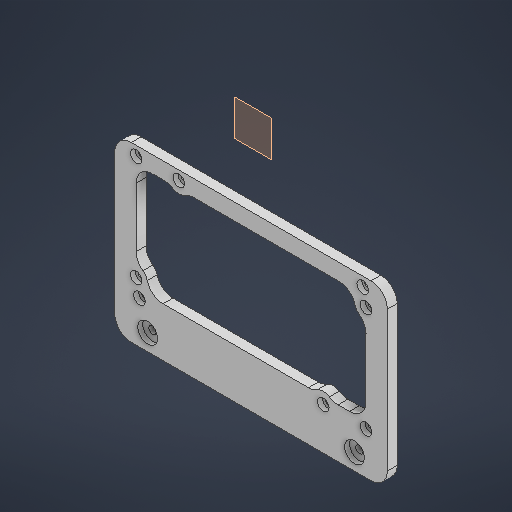
# Autodesk Inventor part: atx_power_holder
Saved by Autodesk Inventor 2026.2 (Build 302298010, 298A)
## iProperties
Created: 2025-02-06
Part Number: atx_power_holder
Material: 一般
Document SubType Name: Modeling
Designer: gisen
Density: 1 g/cm^3
Appearance: 既定
Author: gisen
Autodesk Inventor part; units mm, degrees
ref_plane "YZ Plane" through (0, 0, 0) normal (1, 0, 0) x (0, 1, 0)
ref_plane "XZ Plane" through (0, 0, 0) normal (0, 1, 0) x (-1, 0, 0)
ref_plane "XY Plane" through (0, 0, 0) normal (0, 0, 1) x (1, 0, 0)
sketch "スケッチ1" plane through (0, 0, 0) normal (0, 0, 1) x (1, 0, 0)
  circle A0 centre (44, 4.4) radius 1.25 construction
  circle A1 centre (68, 78.4) radius 1.25 construction
  circle A2 centre (-70, 78.4) radius 1.25 construction
  circle A3 centre (-70, 14.4) radius 1.25 construction
  arc A4 (22.159, 26.4069) -> (22.159, 19.1931) centre (24.5, 22.8) ccw construction
  line L0 (22.159, 26.4069) -> (30.5, 31.8205) construction
  line L1 (30.5, 13.7795) -> (22.159, 19.1931) construction
  line L2 (58.5, 31.8205) -> (66.841, 26.4069) construction
  arc A5 (66.841, 19.1931) -> (66.841, 26.4069) centre (64.5, 22.8) ccw construction
  line L3 (58.5, 13.7795) -> (66.841, 19.1931) construction
  line L4 (35.3264, 11.8) -> (53.6736, 11.8) construction
  line L5 (73.8, 84.2) -> (-73.8, 84.2) construction
  line L6 (75, 83) -> (75, 9.6971) construction
  line L7 (-75, 5.3) -> (-75, 0) construction
  line L8 (75, 0) -> (75, 5.3) construction
  line L9 (-75, 84.2) -> (75, 84.2) construction
  line L10 (75, 84.2) -> (75, -1.2) construction
  line L11 (75, -1.2) -> (-75, -1.2) construction
  line L12 (-75, -1.2) -> (-75, 84.2) construction
  line L13 (-73, -1.2) -> (73, -1.2) construction
  line L14 (75, 84.2) -> (-75, -1.2) construction
  circle A6 centre (-70, 78.4) radius 1.7
  circle A7 centre (-70, 14.4) radius 1.7
  circle A8 centre (44, 4.4) radius 1.7
  circle A9 centre (68, 78.4) radius 1.7
  circle A10 centre (-70, 78.4) radius 7 construction
  circle A11 centre (-70, 14.4) radius 7 construction
  circle A12 centre (44, 4.4) radius 7 construction
  circle A13 centre (68, 78.4) radius 7 construction
  circle A14 centre (70, 4.6) radius 7 construction
  circle A15 centre (70, 4.6) radius 1.7
  circle A16 centre (70, 68.6) radius 7 construction
  circle A17 centre (70, 68.6) radius 1.7
  circle A18 centre (-44, 78.6) radius 7 construction
  circle A19 centre (-44, 78.6) radius 1.7
  circle A20 centre (-68, 4.6) radius 7 construction
  circle A21 centre (-68, 4.6) radius 1.7
  line L15 (-70, 74.2) -> (70, 74.2) construction
  line L16 (70, 74.2) -> (70, 8.8) construction
  line L17 (70, 8.8) -> (-70, 8.8) construction
  line L18 (-70, 8.8) -> (-70, 74.2) construction
  line L19 (90, 128.8) -> (-75, 128.8)
  line L20 (-75, 128.8) -> (-75, -1.2)
  line L21 (-75, -1.2) -> (90, -1.2)
  line L22 (90, -1.2) -> (90, 128.8)
  line L23 (-70, 71.4) -> (-70, 21.4)
  line L24 (-64.4, 74.2) -> (-49.4443, 74.2)
  line L25 (-38.5557, 74.2) -> (62.4, 74.2)
  line L26 (70, 61.6) -> (70, 11.6)
  line L27 (64.4, 8.8) -> (49.4443, 8.8)
  line L28 (38.5557, 8.8) -> (-62.4, 8.8)
  arc A22 (-64.201, 10.4794) -> (-70, 21.4) centre (-70, 14.4) ccw
  arc A23 (-62.4, 8.8) -> (-64.201, 10.4794) centre (-68, 4.6) ccw
  arc A24 (-70, 71.4) -> (-64.4, 74.2) centre (-70, 78.4) ccw
  arc A25 (-49.4443, 74.2) -> (-38.5557, 74.2) centre (-44, 78.6) ccw
  arc A26 (62.4, 74.2) -> (64.201, 72.5206) centre (68, 78.4) ccw
  arc A27 (64.201, 72.5206) -> (70, 61.6) centre (70, 68.6) ccw
  arc A28 (70, 11.6) -> (64.4, 8.8) centre (70, 4.6) ccw
  arc A29 (49.4443, 8.8) -> (38.5557, 8.8) centre (44, 4.4) ccw
  line L29 (-75, 84.2) -> (75, 84.2)
  line L30 (75, 84.2) -> (75, -1.2)
  point P0 (0, 0)
  point P1 (0, 41.5)
  point P2 (90, -1.2)
  point P3 (75, -1.2)
  dimension "d0" = 3.4
  dimension "d1" = 14
  dimension "d4" = 360
  dimension "d6" = 5
  dimension "d7" = 5
  dimension "d8" = 10
  dimension "d9" = 10
  dimension "d10" = 0
  constraints: 42 end point, 32 point on circle, 24 centre point, 21 coincident, 16 point on line, 6 equal radius, 6 parallel, 3 horizontal, 3 perpendicular, 1 midpoint, 35 other
  measures "d0" diameter of A6
  measures "d1" diameter of A10
  measures "d6" distance between parallel lines of L6 L16
  measures "d7" distance between parallel lines of L18 L12
  measures "d8" distance between parallel lines of L13 L17
  measures "d9" distance between parallel lines of L15 L5
  measures "d10" distance between parallel lines of L12 L20
extrude "押し出し1" add sketch "スケッチ1" along normal blind 6 from surface at 0 contours L29 L30 L21 L20
ref_plane "作業平面3" through (1.1555, 128.8, 6) normal (0, 0, 1) x (1, 0, 0)
sketch "スケッチ6" plane through (1.1555, 128.8, 6) normal (0, 0, 1) x (1, 0, 0)
  circle A0 centre (-69.1555, -124.2) radius 1.7 projected
  circle A1 centre (-71.1555, -114.4) radius 1.7 projected
  circle A2 centre (-71.1555, -50.4) radius 1.7 projected
  circle A3 centre (-45.1555, -50.2) radius 1.7 projected
  circle A4 centre (66.8445, -50.4) radius 1.7 projected
  circle A5 centre (68.8445, -60.2) radius 1.7 projected
  circle A6 centre (68.8445, -124.2) radius 1.7 projected
  circle A7 centre (42.8445, -124.4) radius 1.7 projected
  circle A8 centre (-71.1555, -50.4) radius 3.5
  circle A9 centre (-71.1555, -114.4) radius 3.5
  circle A10 centre (-69.1555, -124.2) radius 3.5
  circle A11 centre (-45.1555, -50.2) radius 3.5
  circle A12 centre (66.8445, -50.4) radius 3.5
  circle A13 centre (68.8445, -60.2) radius 3.5
  circle A14 centre (68.8445, -124.2) radius 3.5
  circle A15 centre (42.8445, -124.4) radius 3.5
  point P0 (-1.1555, -128.8)
  dimension "d22" = 7
  constraints: 8 centre point, 8 coincident, 7 equal radius
  measures "d22" diameter of A8
extrude "押し出し5" cut sketch "スケッチ6" along normal blind 10 and the other way blind 3 contours A0 | A1 | A2 | A3 | A4 | A5 | A6 | A7 | A8 | A9 | A10 | A11 | A12 | A13 | A14 | A15
sketch "スケッチ7" plane through (75, -1.2, 0) normal (0, 0, -1) x (-1, 0, 0)
  line L0 (150, 0) -> (150, 85.4) projected
  line L1 (0, 0) -> (150, 0) projected
  line L2 (0, 85.4) -> (0, 0) projected
  line L3 (150, 85.4) -> (158, 85.4)
  line L4 (158, 85.4) -> (158, -20)
  line L5 (158, -20) -> (-8, -20)
  line L6 (-8, -20) -> (-8, 85.4)
  line L7 (-8, 85.4) -> (0, 85.4)
  line L8 (158, -10) -> (-8, -10) construction
  circle A0 centre (12, -10) radius 2.25
  circle A1 centre (138, -10) radius 2.25
  point P0 (75, 1.2)
  dimension "d29" = 20
  dimension "d30" = 8
  dimension "d31" = 10
  dimension "d32" = 4.5
  dimension "d33" = 20
  dimension "d34" = 20
  constraints: 12 end point, 5 point on line, 4 perpendicular, 2 centre point, 2 horizontal, 1 collinear, 1 equal radius
  measures "d29" distance between parallel lines of L5 L1
  measures "d30" distance between parallel lines of L0 L4
  measures "d31" distance between parallel lines of L8 L5
  measures "d32" diameter of A0
  measures "d33" distance from line of A0.centre L6
  measures "d34" distance from line of L4 A1.centre
extrude "押し出し6" add sketch "スケッチ7" against normal up to surface (6 mm away)
fillet "フィレット4" radius 10 14 edges at (62.4, 74.2, 3) (64.201, 72.5206, 3) (70, 61.6, 3) (70, 11.6, 3) (64.4, 8.8, 3) (49.4443, 8.8, 3) (38.5557, 8.8, 3) (-62.4, 8.8, 3) (-64.201, 10.4794, 3) (-70, 21.4, 3) (-70, 71.4, 3) (-64.4, 74.2, 3) (-38.5557, 74.2, 3) (-49.4443, 74.2, 3)
fillet "フィレット5" radius 10 4 edges at (-83, 84.2, 3) (83, 84.2, 3) (83, -21.2, 3) (-83, -21.2, 3)
sketch "スケッチ8" plane through (-73, -21.2, 6) normal (0, 0, 1) x (1, 0, 0)
  circle A0 centre (10, 10) radius 2.25 construction
  circle A1 centre (136, 10) radius 2.25 construction
  circle A2 centre (10, 10) radius 6
  circle A3 centre (136, 10) radius 6
  point P0 (73, 21.2)
  dimension "d39" = 12
  constraints: 2 centre point, 2 coincident, 1 equal radius
  measures "d39" diameter of A2
extrude "押し出し7" cut sketch "スケッチ8" against normal blind 3
equation "\"d7\" = d6"
equation "\"d9\" = d8"
equation "\"d31\" = 0.5 * d29"
equation "\"d34\" = d33"
